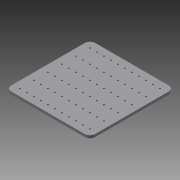
# Autodesk Inventor part: mic6_plate
Saved by Autodesk Inventor 2014 (Build 180170000, 170)
## iProperties
Created: 2014-08-09
Part Number: mic6_plate
Material: Generic
Document SubType Name: Modeling
Designer: Matthew
Density: 1 g/cm^3
Appearance: Default
Author: Matthew
Autodesk Inventor part; units mm, degrees
ref_plane "YZ Plane" through (0, 0, 0) normal (1, 0, 0) x (0, 1, 0)
ref_plane "XZ Plane" through (0, 0, 0) normal (0, 1, 0) x (-1, 0, 0)
ref_plane "XY Plane" through (0, 0, 0) normal (0, 0, 1) x (1, 0, 0)
sketch "Sketch1" plane through (0, 0, 0) normal (0, 1, 0) x (-1, 0, 0)
  line L0 (152.4, 152.4) -> (-152.4, 152.4)
  line L1 (-152.4, 152.4) -> (-152.4, -152.4)
  line L2 (-152.4, -152.4) -> (152.4, -152.4)
  line L3 (152.4, -152.4) -> (152.4, 152.4)
  line L4 (152.4, 152.4) -> (-152.4, -152.4) construction
  line L5 (-152.4, 152.4) -> (152.4, -152.4) construction
  point P0 (0, 0)
  dimension "d0" = 304.8
  dimension "d1" = 304.8
  constraints: 12 end point, 2 midpoint, 2 parallel, 1 horizontal, 1 perpendicular
  measures "d0" distance of L2.end L1.end
  measures "d1" distance of L0.end L1.end
extrude "Extrusion1" add sketch "Sketch1" along normal blind 9.525
fillet "Fillet1" radius 19.05 1 edges at (152.4, 4.7625, 152.4)
fillet "Fillet2" radius 19.05 1 edges at (152.4, 4.7625, -152.4)
fillet "Fillet3" radius 19.05 1 edges at (-152.4, 4.7625, 152.4)
fillet "Fillet4" radius 19.05 1 edges at (-152.4, 4.7625, -152.4)
sketch "Sketch2" plane through (0, 9.525, 0) normal (0, 1, 0) x (1, 0, 0)
  line L0 (-152.4, 133.35) -> (-152.4, -133.35) projected
  line L1 (-133.35, -152.4) -> (133.35, -152.4) projected
  point P0 (0, 0)
  point P1 (-127, -127)
  point P2 (-127, -76.2)
  point P3 (-127, -25.4)
  point P4 (-127, 25.4)
  point P5 (-127, 76.2)
  point P6 (-127, 127)
  point P7 (-101.6, -127)
  point P8 (-101.6, -76.2)
  point P9 (-101.6, -25.4)
  point P10 (-101.6, 25.4)
  point P11 (-101.6, 76.2)
  point P12 (-101.6, 127)
  point P13 (-76.2, -127)
  point P14 (-76.2, -76.2)
  point P15 (-76.2, -25.4)
  point P16 (-76.2, 25.4)
  point P17 (-76.2, 76.2)
  point P18 (-76.2, 127)
  point P19 (-50.8, -127)
  point P20 (-50.8, -76.2)
  point P21 (-50.8, -25.4)
  point P22 (-50.8, 25.4)
  point P23 (-50.8, 76.2)
  point P24 (-50.8, 127)
  point P25 (-25.4, -127)
  point P26 (-25.4, -76.2)
  point P27 (-25.4, -25.4)
  point P28 (-25.4, 25.4)
  point P29 (-25.4, 76.2)
  point P30 (-25.4, 127)
  point P31 (0, -127)
  point P32 (0, -76.2)
  point P33 (0, -25.4)
  point P34 (0, 25.4)
  point P35 (0, 76.2)
  point P36 (0, 127)
  point P37 (25.4, -127)
  point P38 (25.4, -76.2)
  point P39 (25.4, -25.4)
  point P40 (25.4, 25.4)
  point P41 (25.4, 76.2)
  point P42 (25.4, 127)
  point P43 (50.8, -127)
  point P44 (50.8, -76.2)
  point P45 (50.8, -25.4)
  point P46 (50.8, 25.4)
  point P47 (50.8, 76.2)
  point P48 (50.8, 127)
  point P49 (76.2, -127)
  point P50 (76.2, -76.2)
  point P51 (76.2, -25.4)
  point P52 (76.2, 25.4)
  point P53 (76.2, 76.2)
  point P54 (76.2, 127)
  point P55 (101.6, -127)
  point P56 (101.6, -76.2)
  point P57 (101.6, -25.4)
  point P58 (101.6, 25.4)
  point P59 (101.6, 76.2)
  point P60 (101.6, 127)
  point P61 (127, -127)
  point P62 (127, -76.2)
  point P63 (127, -25.4)
  point P64 (127, 25.4)
  point P65 (127, 76.2)
  point P66 (127, 127)
  dimension "d8" = 25.4
  dimension "d9" = 25.4
  dimension "d12" = 50.8
  dimension "d15" = 25.4
  constraints: 1 horizontal, 1 vertical, 65 other
  measures "d8" distance from line of point (-127, -127) L1
  measures "d9" distance from line of L0 point (-127, -127)
  measures "d12" distance of point (-127, -127) point (-127, -76.2)
  measures "d15" distance of point (-127, -127) point (-101.6, -127)
hole "Hole1" at (-127, 9.525, 127) at (-127, 9.525, 76.2) at (-127, 9.525, 25.4) at (-127, 9.525, -25.4) at (-127, 9.525, -76.2) at (-127, 9.525, -127) at (-101.6, 9.525, 127) at (-101.6, 9.525, 76.2) at (-101.6, 9.525, 25.4) at (-101.6, 9.525, -25.4) at (-101.6, 9.525, -76.2) at (-101.6, 9.525, -127) at (-76.2, 9.525, 127) at (-76.2, 9.525, 76.2) at (-76.2, 9.525, 25.4) at (-76.2, 9.525, -25.4) at (-76.2, 9.525, -76.2) at (-76.2, 9.525, -127) at (-50.8, 9.525, 127) at (-50.8, 9.525, 76.2) at (-50.8, 9.525, 25.4) at (-50.8, 9.525, -25.4) at (-50.8, 9.525, -76.2) at (-50.8, 9.525, -127) at (-25.4, 9.525, 127) at (-25.4, 9.525, 76.2) at (-25.4, 9.525, 25.4) at (-25.4, 9.525, -25.4) at (-25.4, 9.525, -76.2) at (-25.4, 9.525, -127) at (0, 9.525, 127) at (0, 9.525, 76.2) at (0, 9.525, 25.4) at (0, 9.525, -25.4) at (0, 9.525, -76.2) at (0, 9.525, -127) at (25.4, 9.525, 127) at (25.4, 9.525, 76.2) at (25.4, 9.525, 25.4) at (25.4, 9.525, -25.4) at (25.4, 9.525, -76.2) at (25.4, 9.525, -127) at (50.8, 9.525, 127) at (50.8, 9.525, 76.2) at (50.8, 9.525, 25.4) at (50.8, 9.525, -25.4) at (50.8, 9.525, -76.2) at (50.8, 9.525, -127) at (76.2, 9.525, 127) at (76.2, 9.525, 76.2) direction (0, -1, 0) diameter 5.842 depth 25.4 tip angle 118 and at (76.2, 9.525, 25.4) (76.2, 9.525, -25.4) (76.2, 9.525, -76.2) (76.2, 9.525, -127) (101.6, 9.525, 127) (101.6, 9.525, 76.2) (101.6, 9.525, 25.4) (101.6, 9.525, -25.4) (101.6, 9.525, -76.2) (101.6, 9.525, -127) (127, 9.525, 127) (127, 9.525, 76.2) (127, 9.525, 25.4) (127, 9.525, -25.4) (127, 9.525, -76.2) (127, 9.525, -127)
body "Solid1"
